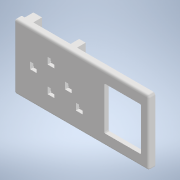
# Autodesk Inventor part: Upper_Half
Saved by Autodesk Inventor 2022 (Build 260153000, 153)
## iProperties
Created: 2023-09-02
Part Number: Upper_Half
Material: Generic
Document SubType Name: Modeling
Designer: Petr Černý
Density: 1 g/cm^3
Appearance: Default
Author: Petr Černý
Autodesk Inventor part; units mm, degrees
ref_plane "YZ Plane" through (0, 0, 0) normal (1, 0, 0) x (0, 1, 0)
ref_plane "XZ Plane" through (0, 0, 0) normal (0, 1, 0) x (-1, 0, 0)
ref_plane "XY Plane" through (0, 0, 0) normal (0, 0, 1) x (1, 0, 0)
sketch "Sketch1" plane through (0, 0, 0) normal (0, 0, 1) x (1, 0, 0)
  line L0 (110.9399, 39.6241) -> (-14.0601, 39.6241)
  line L1 (-14.0601, 39.6241) -> (-14.0601, -20.3759)
  line L2 (-14.0601, -20.3759) -> (110.9399, -20.3759)
  line L3 (110.9399, -20.3759) -> (110.9399, 39.6241)
  point P0 (0, 0)
  dimension "d0" = 125
  dimension "d1" = 60
  constraints: 8 end point, 2 parallel, 1 horizontal, 1 perpendicular
  measures "d0" distance of L1.end L2.end
  measures "d1" distance of L0.end L1.end
extrude "Extrusion1" add sketch "Sketch1" along normal blind 6
shell "Shell1" thickness 2 removed faces 1 at (27.6065, 19.6241, 0)
sketch "Sketch5" plane through (108.9399, -18.3759, 4) normal (0, 0, -1) x (-1, 0, 0)
  line L0 (0, 0) -> (0, 56) projected
  line L1 (0, 0) -> (46.7, 0)
  line L2 (0, 51) -> (0, 0)
  line L3 (0, 0) -> (0, 56) projected
  line L4 (0, 2.5) -> (46.7, 2.5)
  line L5 (46.7, 2.5) -> (46.7, 53.5)
  line L6 (46.7, 53.5) -> (0, 53.5)
  line L7 (0, 53.5) -> (0, 2.5)
  line L8 (0, 56) -> (121, 56) projected
  point P0 (108.9399, 18.3759)
  point P1 (0, 53.5)
  dimension "d124" = 46.7
  dimension "d125" = 51
  dimension "d126" = 2.5
  constraints: 12 end point, 2 horizontal, 2 parallel, 1 perpendicular, 1 point on line
  measures "d124" distance of L6.end L5.end
  measures "d125" distance of L5.end L4.end
  measures "d126" distance between parallel lines of L6 L8
extrude "Extrusion3" add sketch "Sketch5" along normal blind 2
sketch "Sketch6" plane through (108.9399, -18.3759, 2) normal (0, 0, -1) x (-1, 0, 0)
  line L0 (5.2, 8.05) -> (39.2, 8.05)
  line L1 (39.2, 8.05) -> (39.2, 47.95)
  line L2 (39.2, 47.95) -> (5.2, 47.95)
  line L3 (5.2, 47.95) -> (5.2, 8.05)
  line L4 (0, 0) -> (0, 56) projected
  line L5 (121, 0) -> (0, 0) projected
  line L6 (0, 56) -> (121, 56) projected
  point P0 (108.9399, 18.3759)
  point P1 (72, 0)
  point P2 (72, 56)
  dimension "d60" = 34
  dimension "d61" = 39.9
  dimension "d62" = 8.05
  dimension "d63" = 5.2
  constraints: 8 end point, 2 parallel, 1 horizontal, 1 perpendicular
  measures "d60" distance of L2.end L1.end
  measures "d61" distance of L1.end L0.end
  measures "d62" distance between parallel lines of L5 L0
  measures "d63" distance between parallel lines of L3 L4
extrude "Extrusion4" cut sketch "Sketch6" against normal through all
fillet "Fillet1" radius 2 8 edges at (-14.0601, 9.6241, 6) (48.4399, -20.3759, 6) (110.9399, 9.6241, 6) (48.4399, 39.6241, 6) (-14.0601, -20.3759, 3) (-14.0601, 39.6241, 3) (110.9399, -20.3759, 3) (110.9399, 39.6241, 3)
fillet "Fillet2" radius 1 4 edges at (103.7399, 29.5741, 4) (69.7399, 29.5741, 4) (69.7399, -10.3259, 4) (103.7399, -10.3259, 4)
fillet "Fillet7" radius 2 2 edges at (108.9399, 37.6241, 2) (108.9399, -18.3759, 2)
sketch "Sketch11" plane through (-12.0601, -18.3759, 4) normal (0, 0, -1) x (-1, 0, 0)
  line L0 (0, 56) -> (-121, 56) projected
  line L1 (0, 56) -> (-8, 56)
  line L2 (-8, 56) -> (-8, 48)
  line L3 (-8, 48) -> (0, 48)
  line L4 (0, 48) -> (0, 56)
  line L5 (-42.5, 56) -> (-48.5, 56)
  line L6 (-48.5, 56) -> (-48.5, 48)
  line L7 (-48.5, 48) -> (-42.5, 48)
  line L8 (-42.5, 48) -> (-42.5, 56)
  line L9 (0, 0) -> (-119, 0) projected
  line L10 (-48.5, 0) -> (-42.5, 0)
  line L11 (-42.5, 0) -> (-42.5, 13)
  line L12 (-42.5, 13) -> (-48.5, 13)
  line L13 (-48.5, 13) -> (-48.5, 0)
  line L14 (0, 0) -> (-8, 0)
  line L15 (-8, 0) -> (-8, 12)
  line L16 (-8, 12) -> (0, 12)
  line L17 (0, 12) -> (0, 0)
  point P0 (-12.0601, 18.3759)
  point P1 (-42.5, 0)
  dimension "d127" = 8
  dimension "d128" = 8
  dimension "d129" = 6
  dimension "d130" = 8
  dimension "d131" = 6
  dimension "d132" = 13
  dimension "d133" = 8
  dimension "d134" = 12
  dimension "d135" = 34.5
  dimension "d136" = 34.5
  constraints: 32 end point, 8 parallel, 4 horizontal, 4 perpendicular, 2 point on line
  measures "d127" distance of L3.end L2.end
  measures "d128" distance of L2.end L1.end
  measures "d129" distance of L7.end L6.end
  measures "d130" distance of L6.end L5.end
  measures "d131" distance of L12.end L11.end
  measures "d132" distance of L11.end L10.end
  measures "d133" distance of L15.end L16.end
  measures "d134" distance of L14.end L15.end
  measures "d135" distance between parallel lines of L8 L2
  measures "d136" distance between parallel lines of L11 L15
extrude "Extrusion7" add sketch "Sketch11" along normal blind 14
sketch "Sketch12" plane through (-12.0601, -18.3759, -10) normal (0, 0, -1) x (-1, 0, 0)
  circle A0 centre (-5, 51.5) radius 1.5 projected
  circle A1 centre (-5, 9.4) radius 1.5 projected
  circle A2 centre (-45, 9.4) radius 1.5 projected
  circle A3 centre (-45, 51.55) radius 1.6 projected
  point P0 (-12.0601, 18.3759)
  constraints: 4 coincident
hole "Hole4" at (32.9399, 33.1741, -10) at (32.9399, -8.9759, -10) at (-7.0601, -8.9759, -10) at (-7.0601, 33.1241, -10) direction (0, 0, 1) diameter 2.459 depth 8.8 tip angle 118 thread size "M3x0.5" class "6H" standard "ISO Metric profile"
sketch "Sketch14" plane through (108.9399, 35.1241, 4) normal (0, 0, -1) x (-1, 0, 0)
  line L0 (2, 2.5) -> (72.5, 2.5) projected
  circle A0 centre (76, -1.95) radius 1.2295 projected
  line L1 (78.5, -5.5) -> (78.5, 2.5) projected
  line L2 (78.5, 2.5) -> (72.5, 2.5) projected
  line L3 (72.5, 2.5) -> (72.5, -5.5) projected
  line L4 (72.5, -5.5) -> (78.5, -5.5) projected
  circle A1 centre (116, -2) radius 1.2295 projected
  line L5 (121, 2.5) -> (113, 2.5) projected
  line L6 (113, 2.5) -> (113, -5.5) projected
  line L7 (113, -5.5) -> (121, -5.5) projected
  line L8 (121, -5.5) -> (121, 2.5) projected
  line L9 (78.5, 2.5) -> (113, 2.5) projected
  line L10 (121, -5.5) -> (121, -41.5) projected
  circle A2 centre (116, -44.1) radius 1.2295 projected
  line L11 (121, -41.5) -> (113, -41.5) projected
  line L12 (113, -41.5) -> (113, -53.5) projected
  line L13 (113, -53.5) -> (121, -53.5) projected
  line L14 (121, -53.5) -> (121, -41.5) projected
  line L15 (113, -53.5) -> (78.5, -53.5) projected
  circle A3 centre (76, -44.1) radius 1.2295 projected
  line L16 (72.5, -40.5) -> (72.5, -53.5) projected
  line L17 (72.5, -53.5) -> (78.5, -53.5) projected
  line L18 (78.5, -53.5) -> (78.5, -40.5) projected
  line L19 (78.5, -40.5) -> (72.5, -40.5) projected
  line L20 (72.5, -53.5) -> (2, -53.5) projected
  line L21 (0, -51) -> (46.7, -51) projected
  line L22 (46.7, -51) -> (46.7, 0) projected
  line L23 (46.7, 0) -> (0, 0) projected
  line L24 (6.2, -5.55) -> (38.2, -5.55) projected
  arc A4 (39.2, -6.55) -> (38.2, -5.55) centre (38.2, -6.55) ccw projected
  line L25 (39.2, -6.55) -> (39.2, -44.45) projected
  arc A5 (38.2, -45.45) -> (39.2, -44.45) centre (38.2, -44.45) ccw projected
  line L26 (38.2, -45.45) -> (6.2, -45.45) projected
  arc A6 (5.2, -44.45) -> (6.2, -45.45) centre (6.2, -44.45) ccw projected
  line L27 (5.2, -44.45) -> (5.2, -6.55) projected
  arc A7 (6.2, -5.55) -> (5.2, -6.55) centre (6.2, -6.55) ccw projected
  line L28 (0, 0) -> (46.7, 0) projected
  arc A8 (2, 2.5) -> (0, 0.5) centre (2, 0.5) ccw projected
  line L29 (0, 0) -> (0, 0.5)
  arc A9 (2, 2.5) -> (0, 0.5) centre (2, 0.5) ccw
  line L30 (2, 2.5) -> (72.5, 2.5) projected
  line L31 (2, 2.5) -> (72.5, 2.5)
  line L32 (72.5, -5.5) -> (72.5, 2.5) projected
  line L33 (72.5, 2.5) -> (72.5, -5.5)
  line L34 (78.5, -5.5) -> (72.5, -5.5) projected
  line L35 (72.5, -5.5) -> (78.5, -5.5)
  line L36 (78.5, 2.5) -> (78.5, -5.5) projected
  line L37 (78.5, -5.5) -> (78.5, 2.5)
  line L38 (78.5, 2.5) -> (113, 2.5)
  line L39 (113, -5.5) -> (113, 2.5) projected
  line L40 (121, -5.5) -> (113, -5.5) projected
  line L41 (113, -5.5) -> (121, -5.5)
  line L42 (113, -41.5) -> (121, -41.5) projected
  line L43 (121, -5.5) -> (121, -41.5)
  line L44 (121, -41.5) -> (113, -41.5)
  line L45 (113, -53.5) -> (113, -41.5) projected
  line L46 (113, -53.5) -> (78.5, -53.5)
  line L47 (78.5, -40.5) -> (78.5, -53.5) projected
  line L48 (72.5, -40.5) -> (78.5, -40.5) projected
  line L49 (78.5, -40.5) -> (72.5, -40.5)
  line L50 (72.5, -53.5) -> (72.5, -40.5) projected
  line L51 (72.5, -40.5) -> (72.5, -53.5)
  arc A10 (0, -51.5) -> (2, -53.5) centre (2, -51.5) ccw projected
  line L52 (72.5, -53.5) -> (2, -53.5)
  arc A11 (0, -51) -> (2, -53.5) centre (2, -51.45) ccw
  line L53 (46.7, -51) -> (0, -51) projected
  line L54 (0, -51) -> (46.7, -51)
  line L55 (46.7, 0) -> (46.7, -51) projected
  line L56 (46.7, -51) -> (46.7, 0)
  line L57 (0, 0) -> (0, 0.5) projected
  line L58 (46.7, 0) -> (0, 0)
  line L59 (0, -51) -> (0, 0) projected
  point P0 (108.9399, -35.1241)
  point P1 (1, 0)
  point P2 (1, -51)
  point P3 (78.5, -53.5)
  point P4 (72.5, 2.5)
  point P5 (0, -51)
  constraints: 32 end point, 12 perpendicular, 5 tangent, 4 point on circle, 2 centre point, 2 horizontal, 1 collinear, 1 point on line, 1 vertical
extrude "Extrusion9" add sketch "Sketch14" along normal blind 2 contours L0 L3 L4 L1 L9 L6 L7 L10 L11 L12 L15 L18 L19 L16 L20 A11 L21 L22 L23 L29 A8
sketch "Sketch15" plane through (0, 0, 6) normal (0, 0, 1) x (1, 0, 0)
  line L0 (7.1399, 12.7241) -> (0.9399, 12.7241)
  line L1 (0.9399, 12.7241) -> (0.9399, 6.5241)
  line L2 (0.9399, 6.5241) -> (7.1399, 6.5241)
  line L3 (7.1399, 6.5241) -> (7.1399, 12.7241)
  line L4 (23.3399, 24.6241) -> (17.1399, 24.6241)
  line L5 (17.1399, 24.6241) -> (17.1399, 18.4241)
  line L6 (17.1399, 18.4241) -> (23.3399, 18.4241)
  line L7 (23.3399, 18.4241) -> (23.3399, 24.6241)
  line L8 (23.3399, 0.8241) -> (17.1399, 0.8241)
  line L9 (17.1399, 0.8241) -> (17.1399, -5.3759)
  line L10 (17.1399, -5.3759) -> (23.3399, -5.3759)
  line L11 (23.3399, -5.3759) -> (23.3399, 0.8241)
  line L12 (39.5399, 12.7241) -> (33.3399, 12.7241)
  line L13 (33.3399, 12.7241) -> (33.3399, 6.5241)
  line L14 (33.3399, 6.5241) -> (39.5399, 6.5241)
  line L15 (39.5399, 6.5241) -> (39.5399, 12.7241)
  line L16 (49.5399, 0.8241) -> (43.3399, 0.8241)
  line L17 (43.3399, 0.8241) -> (43.3399, -5.3759)
  line L18 (43.3399, -5.3759) -> (49.5399, -5.3759)
  line L19 (49.5399, -5.3759) -> (49.5399, 0.8241)
  line L20 (-14.0601, 37.6241) -> (-14.0601, -18.3759) projected
  line L21 (-12.0601, -20.3759) -> (108.9399, -20.3759) projected
  line L22 (108.9399, 39.6241) -> (-12.0601, 39.6241) projected
  point P0 (0, 0)
  dimension "d170" = 6.2
  dimension "d171" = 6.2
  dimension "d172" = 15
  dimension "d173" = 26.9
  dimension "d174" = 6.2
  dimension "d175" = 6.2
  dimension "d176" = 10
  dimension "d177" = 15
  dimension "d178" = 10
  dimension "d179" = 6.2
  dimension "d180" = 15
  dimension "d181" = 6.2
  dimension "d182" = 6.2
  dimension "d183" = 0
  dimension "d184" = 10
  dimension "d185" = 6.2
  dimension "d186" = 6.2
  dimension "d187" = 20
  constraints: 40 end point, 10 parallel, 5 horizontal, 5 perpendicular, 2 point on line
  measures "d170" distance of L2.end L0.start
  measures "d171" distance of L1.end L2.end
  measures "d172" distance between parallel lines of L1 L20
  measures "d173" distance between parallel lines of L2 L21
  measures "d174" distance of L4.end L5.end
  measures "d175" distance of L4.start L4.end
  measures "d176" distance between parallel lines of L5 L3
  measures "d177" distance between parallel lines of L22 L4
  measures "d178" distance between parallel lines of L9 L3
  measures "d179" distance of L10.end L8.start
  measures "d180" distance between parallel lines of L21 L10
  measures "d181" distance of L14.end L12.start
  measures "d182" distance of L12.start L12.end
  measures "d183" distance between parallel lines of L0 L12
  measures "d184" distance between parallel lines of L13 L7
  measures "d185" distance of L16.end L17.end
  measures "d186" distance of L17.end L18.end
  measures "d187" distance between parallel lines of L17 L11
extrude "Extrusion10" cut sketch "Sketch15" against normal blind 3
sketch "Sketch16" plane through (0, 0, 3) normal (0, 0, 1) x (1, 0, 0)
  line L0 (0.9399, 6.5241) -> (0.9399, 12.7241) projected
  line L1 (7.1399, 6.5241) -> (0.9399, 6.5241) projected
  line L2 (7.1399, 12.7241) -> (7.1399, 6.5241) projected
  line L3 (0.9399, 12.7241) -> (7.1399, 12.7241) projected
  line L4 (0.9399, 12.7241) -> (7.1399, 12.7241) projected
  line L5 (4.0399, 12.7241) -> (4.0399, 6.5241)
  line L6 (7.1399, 6.5241) -> (0.9399, 6.5241) projected
  line L7 (0.9399, 6.5241) -> (0.9399, 12.7241) projected
  line L8 (0.9399, 9.6241) -> (7.1399, 9.6241)
  line L9 (17.1399, 18.4241) -> (17.1399, 24.6241) projected
  line L10 (23.3399, 18.4241) -> (17.1399, 18.4241) projected
  line L11 (23.3399, 24.6241) -> (23.3399, 18.4241) projected
  line L12 (17.1399, 24.6241) -> (23.3399, 24.6241) projected
  line L13 (17.1399, -5.3759) -> (17.1399, 0.8241) projected
  line L14 (23.3399, -5.3759) -> (17.1399, -5.3759) projected
  line L15 (23.3399, 0.8241) -> (23.3399, -5.3759) projected
  line L16 (17.1399, 0.8241) -> (23.3399, 0.8241) projected
  line L17 (33.3399, 6.5241) -> (33.3399, 12.7241) projected
  line L18 (39.5399, 6.5241) -> (33.3399, 6.5241) projected
  line L19 (39.5399, 12.7241) -> (39.5399, 6.5241) projected
  line L20 (33.3399, 12.7241) -> (39.5399, 12.7241) projected
  line L21 (45.9399, -18.3759) -> (45.9399, 37.6241) projected
  line L22 (17.1399, 24.6241) -> (23.3399, 24.6241) projected
  line L23 (20.2399, 24.6241) -> (20.2399, 18.4241)
  line L24 (23.3399, 18.4241) -> (17.1399, 18.4241) projected
  line L25 (23.3399, 24.6241) -> (23.3399, 18.4241) projected
  line L26 (23.3399, 21.5241) -> (17.1399, 21.5241)
  line L27 (17.1399, 18.4241) -> (17.1399, 24.6241) projected
  line L28 (17.1399, 0.8241) -> (23.3399, 0.8241) projected
  line L29 (20.2399, 0.8241) -> (20.2399, -5.3759)
  line L30 (23.3399, 0.8241) -> (23.3399, -5.3759) projected
  line L31 (23.3399, -2.2759) -> (17.1399, -2.2759)
  line L32 (17.1399, -5.3759) -> (17.1399, 0.8241) projected
  line L33 (33.3399, 12.7241) -> (39.5399, 12.7241) projected
  line L34 (36.4399, 12.7241) -> (36.4399, 6.5241)
  line L35 (39.5399, 6.5241) -> (33.3399, 6.5241) projected
  line L36 (39.5399, 12.7241) -> (39.5399, 6.5241) projected
  line L37 (39.5399, 9.6241) -> (33.3399, 9.6241)
  line L38 (43.3399, -5.3759) -> (43.3399, 0.8241) projected
  line L39 (49.5399, -5.3759) -> (43.3399, -5.3759) projected
  line L40 (49.5399, 0.8241) -> (49.5399, -5.3759) projected
  line L41 (43.3399, 0.8241) -> (49.5399, 0.8241) projected
  line L42 (43.3399, 0.8241) -> (49.5399, 0.8241) projected
  line L43 (46.4399, 0.8241) -> (46.4399, -5.3759)
  line L44 (49.5399, -5.3759) -> (43.3399, -5.3759) projected
  line L45 (49.5399, 0.8241) -> (49.5399, -5.3759) projected
  line L46 (49.5399, -2.2759) -> (43.3399, -2.2759)
  point P0 (0, 0)
  point P1 (7.2899, 11.8741)
  point P2 (7.2899, 7.3741)
  point P3 (0.7899, 11.8741)
  point P4 (0.7899, 7.3741)
  point P5 (23.4899, 23.7741)
  point P6 (23.4899, 19.2741)
  point P7 (16.9899, 23.7741)
  point P8 (16.9899, 19.2741)
  point P9 (23.4899, -0.0259)
  point P10 (23.4899, -4.5259)
  point P11 (16.9899, -0.0259)
  point P12 (16.9899, -4.5259)
  point P13 (39.6899, 11.8741)
  point P14 (39.6899, 7.3741)
  point P15 (33.1899, 11.8741)
  point P16 (33.1899, 7.3741)
  point P17 (49.6899, -0.0259)
  point P18 (49.6899, -4.5259)
  point P19 (43.1899, -0.0259)
  point P20 (43.1899, -4.5259)
  dimension "d190" = 2.25
  dimension "d191" = 2.25
  dimension "d192" = 3.25
  dimension "d193" = 3.25
  dimension "d194" = 6.5
  dimension "d195" = 6.5
  dimension "d196" = 2.25
  dimension "d197" = 2.25
  dimension "d198" = 2.25
  dimension "d199" = 2.25
  dimension "d200" = 2.25
  dimension "d201" = 2.25
  dimension "d202" = 3.25
  dimension "d203" = 3.25
  dimension "d204" = 3.25
  dimension "d205" = 3.25
  dimension "d206" = 2.25
  dimension "d207" = 2.25
  dimension "d208" = 2.25
  dimension "d209" = 2.25
  dimension "d210" = 3.25
  dimension "d211" = 3.25
  dimension "d212" = 3.25
  dimension "d213" = 3.25
  dimension "d214" = 2.25
  dimension "d215" = 2.25
  dimension "d216" = 2.25
  dimension "d217" = 2.25
  dimension "d218" = 3.25
  dimension "d219" = 3.25
  dimension "d220" = 3.25
  dimension "d221" = 3.25
  dimension "d222" = 2.25
  dimension "d223" = 2.25
  dimension "d224" = 2.25
  dimension "d225" = 2.25
  dimension "d226" = 3.25
  dimension "d227" = 3.25
  dimension "d228" = 3.25
  dimension "d229" = 3.25
  constraints: 20 end point, 20 midpoint
  measures "d190" distance from line of point (7.29, 7.374) L8
  measures "d191" distance from line of point (7.29, 11.874) L8
  measures "d192" distance from line of point (7.29, 11.874) L5
  measures "d193" distance from line of point (7.29, 7.374) L5
  measures "d194" distance of point (0.79, 7.374) point (7.29, 7.374)
  measures "d195" distance of point (0.79, 11.874) point (7.29, 11.874)
  measures "d196" distance from line of L8 point (0.79, 11.874)
  measures "d197" distance from line of point (0.79, 7.374) L8
  measures "d198" distance from line of point (23.49, 23.774) L26
  measures "d199" distance from line of point (23.49, 19.274) L26
  measures "d200" distance from line of point (16.99, 23.774) L26
  measures "d201" distance from line of point (16.99, 19.274) L26
  measures "d202" distance from line of point (23.49, 19.274) L23
  measures "d203" distance from line of point (23.49, 23.774) L23
  measures "d204" distance from line of point (16.99, 23.774) L23
  measures "d205" distance from line of point (16.99, 19.274) L23
  measures "d206" distance from line of point (23.49, -0.026) L31
  measures "d207" distance from line of point (23.49, -4.526) L31
  measures "d208" distance from line of point (16.99, -0.026) L31
  measures "d209" distance from line of point (16.99, -4.526) L31
  measures "d210" distance from line of point (23.49, -4.526) L29
  measures "d211" distance from line of point (23.49, -0.026) L29
  measures "d212" distance from line of point (16.99, -0.026) L29
  measures "d213" distance from line of L29 point (16.99, -4.526)
  measures "d214" distance from line of point (39.69, 11.874) L37
  measures "d215" distance from line of point (39.69, 7.374) L37
  measures "d216" distance from line of point (33.19, 11.874) L37
  measures "d217" distance from line of point (33.19, 7.374) L37
  measures "d218" distance from line of point (33.19, 7.374) L34
  measures "d219" distance from line of point (39.69, 7.374) L34
  measures "d220" distance from line of point (39.69, 11.874) L34
  measures "d221" distance from line of point (33.19, 11.874) L34
  measures "d222" distance from line of point (49.69, -0.026) L46
  measures "d223" distance from line of point (49.69, -4.526) L46
  measures "d224" distance from line of point (43.19, -0.026) L46
  measures "d225" distance from line of point (43.19, -4.526) L46
  measures "d226" distance from line of point (49.69, -0.026) L43
  measures "d227" distance from line of point (49.69, -4.526) L43
  measures "d228" distance from line of point (43.19, -0.026) L43
  measures "d229" distance from line of point (43.19, -4.526) L43
hole "Hole5" at (7.2899, 11.8741, 3) at (7.2899, 7.3741, 3) at (0.7899, 11.8741, 3) at (0.7899, 7.3741, 3) at (23.4899, 23.7741, 3) at (23.4899, 19.2741, 3) at (16.9899, 23.7741, 3) at (16.9899, 19.2741, 3) at (23.4899, -0.0259, 3) at (23.4899, -4.5259, 3) at (16.9899, -0.0259, 3) at (16.9899, -4.5259, 3) at (39.6899, 11.8741, 3) at (39.6899, 7.3741, 3) at (33.1899, 11.8741, 3) at (33.1899, 7.3741, 3) at (49.6899, -0.0259, 3) at (49.6899, -4.5259, 3) at (43.1899, -0.0259, 3) at (43.1899, -4.5259, 3) direction (0, 0, -1) diameter 1 depth 2
body "Solid1"
